rachat tourk (Autodesk Fusion 360 design; units mm, degrees)
Autodesk Fusion 360 part; units mm, degrees
note: some values were not read from the file. Set by a fixed rule: which sketch regions a step uses.
sketch "Sketch1" plane through (0, 0, 0) normal (0, 0, 1) x (1, 0, 0)
  line L0 (26.0398, -10.2827) -> (28.8703, 61.0109)
  line L1 (28.8703, 61.0109) -> (44.8656, 60.6138)
  line L2 (44.8656, 60.6138) -> (42.0951, -11.3634)
  arc A0 (42.0951, -11.3634) -> (46.8265, -28.3625) centre (71.0004, -12.476) ccw
  arc A1 (19.3322, -28.7202) -> (26.0398, -10.2827) centre (-6.169, -9.0039) ccw
  line L3 (19.3322, -28.7202) -> (19.3322, -41.5929)
  arc A2 (19.3322, -41.5929) -> (46.3862, -42.0287) centre (32.8627, -41.5929) ccw
  line L4 (46.3862, -42.0287) -> (46.8265, -28.3625)
  line L5 (32.1606, -39.3761) -> (38.4606, -39.3761)
  line L6 (38.4606, -39.3761) -> (38.4606, -45.6761)
  line L7 (38.4606, -45.6761) -> (32.1606, -45.6761)
  line L8 (32.1606, -45.6761) -> (32.1606, -39.3761)
  line L9 (38.4606, -39.3761) -> (32.1606, -45.6761) construction
  line L10 (32.1606, -39.3761) -> (38.4606, -45.6761) construction
  point P0 (35.3106, -42.5261)
  dimension "d2" = 6.3
  dimension "d3" = 6.3
  constraint tangent L2 A0
  constraint tangent L0 A1
  constraint vertical L3
  constraint tangent L3 A2
  constraint tangent A2 L4
  constraint horizontal L5
  constraint vertical L6
  constraint horizontal L7
  constraint vertical L8
  constraint midpoint L9 P0
  measures "d2" distance of L5.end L6.end
  measures "d3" distance of L5.start L5.end
extrude "Extrude1" add sketch "Sketch1" against normal blind 13.094 contours L0 L1 L2 A0 A1 L3 A2 L4 | L5 L6 L7 L8
extrude "Extrude2" add sketch "Sketch1" along normal blind 5.15 contours L5 L6 L7 L8
equation "d3 = d2"
